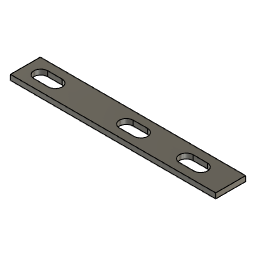
SteCam (Autodesk Fusion 360 design; units mm, degrees)
Autodesk Fusion 360 part; units mm, degrees
sketch "スケッチ1" plane through (0, 0, 0) normal (0, 0, 1) x (1, 0, 0)
  line L0 (120, -17.5) -> (-120, -17.5)
  line L1 (-120, -17.5) -> (-120, 17.5)
  line L2 (-120, 17.5) -> (120, 17.5)
  line L3 (120, 17.5) -> (120, -17.5)
  line L4 (120, -17.5) -> (-120, 17.5) construction
  line L5 (-120, -17.5) -> (120, 17.5) construction
  circle A0 centre (-102, 0) radius 8
  circle A1 centre (-2, 0) radius 8
  circle A2 centre (15, 0) radius 8
  line L6 (-2, -8) -> (15, -8)
  line L7 (-2, 8) -> (15, 8)
  circle A3 centre (68, 0) radius 8
  circle A4 centre (85, 0) radius 8
  line L8 (68.0795, 7.9996) -> (84.9998, 8)
  line L9 (84.9998, -8) -> (68, -8)
  circle A5 centre (-85, 0) radius 8
  line L10 (-102, 8) -> (-85, 8)
  line L11 (-102, -8) -> (-85, -8)
  point P0 (-110, 0)
  point P1 (-102, 0)
  point P2 (-94, 0)
  point P3 (-102, 8)
  point P4 (-10, 0)
  point P5 (23, 0)
  point P6 (-2, 0)
  point P7 (15, 0)
  point P8 (60, 0)
  point P9 (68, 0)
  point P10 (85, 0)
  point P11 (93, 0)
  point P12 (-77, 0)
  point P13 (-85, 0)
  dimension "d1" = 240
  dimension "d2" = 35
  dimension "d3" = 10
  dimension "d4" = 8
  dimension "d5" = 16
  dimension "d8" = 100
  dimension "d9" = 33
  dimension "d10" = 8
  dimension "d11" = 16
  dimension "d12" = 8
  dimension "d13" = 16
  dimension "d14" = 70
  dimension "d15" = 8
  dimension "d16" = 16
  dimension "d17" = 33
  dimension "d18" = 8
  dimension "d19" = 16
  dimension "d20" = 33
  dimension "d21" = 8
  dimension "d22" = 16
  dimension "d23" = 27
  constraint perpendicular L0 L1
  constraint parallel L0 L2
  constraint parallel L1 L3
  constraint horizontal L0
  constraint coincident L4 origin
  constraint coincident L5 origin
  constraint coincident P1 A0.centre
  constraint coincident P2 A0
  constraint coincident P6 A1.centre
  constraint coincident P7 A2.centre
  constraint coincident A1 L6.start
  constraint coincident A2 L6.end
  constraint tangent A2 L6
  constraint horizontal L6
  constraint coincident A1 L7.start
  constraint coincident A2 L7.end
  constraint tangent A2 L7
  constraint parallel L6 L7
  constraint coincident P9 A3.centre
  constraint coincident P10 A4.centre
  constraint coincident A3 L8.start
  constraint coincident A4 L8.end
  constraint tangent A4 L8
  constraint coincident A4 L9.start
  constraint coincident A3 L9.end
  constraint tangent A3 L9
  constraint coincident P13 A5.centre
  constraint coincident P3 L10.start
  constraint coincident A5 L10.end
  constraint tangent A5 L10
  constraint coincident A0 L11.start
  constraint coincident A5 L11.end
  constraint tangent A5 L11
  constraint horizontal L11
  measures "d1" distance of L1.end L2.end
  measures "d2" distance of L0.end L1.end
  measures "d3" distance of L1 P0
  measures "d4" distance of P0 P1
  measures "d5" diameter of A0
  measures "d8" distance of P0 P4
  measures "d9" distance of P4 P5
  measures "d10" distance of P4 P6
  measures "d11" diameter of A1
  measures "d12" distance of P5 P7
  measures "d13" diameter of A2
  measures "d14" distance of P4 P8
  measures "d15" distance of P8 P9
  measures "d16" diameter of A3
  measures "d17" distance of P8 P11
  measures "d18" distance of P10 P11
  measures "d19" diameter of A4
  measures "d20" distance of P0 P12
  measures "d21" distance of P12 P13
  measures "d22" diameter of A5
  measures "d23" distance of L3 P11
extrude "押し出し1" add sketch "スケッチ1" along normal blind 6
